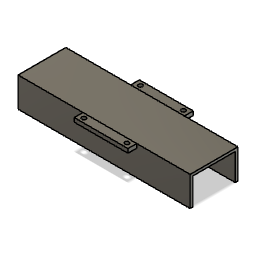
Magnet_Storage_Cover (Autodesk Fusion 360 design; units mm, degrees)
Autodesk Fusion 360 part; units mm, degrees
sketch "base" plane through (0, 0, 0) normal (0, 1, 0) x (1, 0, 0)
  line L0 (-67, 15.5) -> (67, 15.5) construction
  line L1 (67, 15.5) -> (67, -15.5) construction
  line L2 (67, -15.5) -> (-67, -15.5) construction
  line L3 (-67, -15.5) -> (-67, 15.5) construction
  line L4 (0, 15.5) -> (0, -15.5) construction
  line L5 (-67, 0) -> (67, 0) construction
  line L6 (-69.25, 17.75) -> (58.75, 17.75)
  line L7 (58.75, 17.75) -> (58.75, 15.75)
  line L8 (58.75, 15.75) -> (-69.25, 15.75)
  line L9 (-69.25, 15.75) -> (-69.25, 17.75)
  line L10 (-69.25, -15.75) -> (58.75, -15.75)
  line L11 (58.75, -15.75) -> (58.75, -17.75)
  line L12 (58.75, -17.75) -> (-69.25, -17.75)
  line L13 (-69.25, -17.75) -> (-69.25, -15.75)
  line L14 (-69.25, 15.75) -> (-69.25, -15.75)
  line L15 (-67.25, -15.75) -> (-67.25, 15.75)
  dimension "d1" = 134
  dimension "d2" = 31
  dimension "d3" = 128
  dimension "d4" = 2
  dimension "d5" = 2
  dimension "margin" = 0.25
  dimension "d7" = 0.25
  dimension "d8" = 0.25
  constraint horizontal L0
  constraint vertical L1
  constraint horizontal L2
  constraint vertical L3
  constraint midpoint L0 L4.start
  constraint midpoint L2 L4.end
  constraint midpoint L3 L5.start
  constraint midpoint L1 L5.end
  constraint coincident origin L5
  constraint coincident origin L4
  constraint horizontal L6
  constraint vertical L7
  constraint horizontal L8
  constraint vertical L9
  constraint horizontal L10
  constraint vertical L11
  constraint horizontal L12
  constraint vertical L13
  constraint collinear L7 L11
  constraint collinear L9 L13
  constraint coincident L10 L15.start
  constraint coincident L8 L15.end
  constraint perpendicular L8 L15
  constraint equal L9 L13
  measures "d1" distance of L0.start L0.end
  measures "d2" distance of L0.start L2.end
  measures "d3" distance of L6.start L6.end
  measures "d4" distance of L6.start L8.end
  measures "d5" distance of L14 L15
  measures "margin" distance of L3 L15
  measures "d7" distance of L2 L10
  measures "d8" distance of L0 L8
extrude "Extrude1" add sketch "base" along normal blind 20 makes body 1
sketch "top" plane through (0, 20, 0) normal (0, 1, 0) x (-1, 0, 0)
  line L0 (-58.75, 15.75) -> (67.25, 15.75)
  line L1 (67.25, 15.75) -> (67.25, -15.75)
  line L2 (67.25, -15.75) -> (-58.75, -15.75)
  line L3 (-58.75, -15.75) -> (-58.75, -17.75)
  line L4 (-58.75, -17.75) -> (69.25, -17.75)
  line L5 (69.25, -17.75) -> (69.25, 17.75)
  line L6 (69.25, 17.75) -> (-58.75, 17.75)
  line L7 (-58.75, 17.75) -> (-58.75, 15.75)
  line L8 (69.25, -17.75) -> (-58.75, -17.75)
  line L9 (-58.75, -17.75) -> (-58.75, 17.75)
  line L10 (-58.75, 17.75) -> (69.25, 17.75)
  line L11 (69.25, 17.75) -> (69.25, -17.75)
  constraint horizontal L8
  constraint vertical L9
  constraint horizontal L10
  constraint vertical L11
  constraint collinear L3 L9
  constraint collinear L5 L11
  constraint collinear L4 L8
  constraint collinear L6 L10
extrude "Extrude2" add sketch "top" along normal blind 2 bodies 1
sketch "wing supports" plane through (0, 22, 0) normal (0, 1, 0) x (-1, 0, 0)
  line L0 (69.25, 17.75) -> (-58.75, 17.75)
  line L1 (-58.75, 17.75) -> (-58.75, -17.75)
  line L2 (-58.75, -17.75) -> (69.25, -17.75)
  line L3 (69.25, -17.75) -> (69.25, 17.75)
  line L4 (21, -24.25) -> (-19, -24.25)
  line L5 (-19, -24.25) -> (-19, -17.75)
  line L6 (-19, -17.75) -> (21, -17.75)
  line L7 (21, -17.75) -> (21, -24.25)
  line L8 (21, 17.75) -> (-19, 17.75)
  line L9 (-19, 17.75) -> (-19, 24.25)
  line L10 (-19, 24.25) -> (21, 24.25)
  line L11 (21, 24.25) -> (21, 17.75)
  circle A0 centre (17, 21) radius 1.55
  circle A1 centre (-15, 21) radius 1.55
  line L12 (17, 21) -> (-15, 21) construction
  circle A2 centre (17, -21) radius 1.55
  circle A3 centre (-15, -21) radius 1.55
  line L13 (17, -21) -> (-15, -21) construction
  circle A4 centre (17, 21) radius 2.75
  circle A5 centre (-15, 21) radius 2.75
  circle A6 centre (17, -21) radius 2.75
  circle A7 centre (-15, -21) radius 2.75
  dimension "d13" = 6.5
  dimension "d14" = 40
  dimension "d15" = 19
  dimension "d16" = 3.1
  dimension "d17" = 3.25
  dimension "d18" = 4
  dimension "d19" = 4
  dimension "d20" = 3.25
  dimension "d21" = 4
  dimension "d22" = 4
  dimension "d25" = 5.5
  constraint horizontal L4
  constraint vertical L5
  constraint horizontal L6
  constraint vertical L7
  constraint horizontal L8
  constraint vertical L9
  constraint horizontal L10
  constraint vertical L11
  constraint collinear L5 L9
  constraint collinear L7 L11
  constraint collinear L2 L6
  constraint collinear L0 L8
  constraint equal L5 L9
  constraint equal A0 A1
  constraint coincident A0.centre L12.start
  constraint coincident A1.centre L12.end
  constraint horizontal L12
  constraint equal A2 A3
  constraint equal A0 A2
  constraint coincident A2.centre L13.start
  constraint coincident A3.centre L13.end
  constraint parallel L4 L13
  constraint concentric A1 A5
  constraint equal A4 A5
  constraint equal A4 A6
  constraint equal A4 A7
  measures "d13" distance of L4.end L5.end
  measures "d14" distance of L9.end L10.end
  measures "d15" distance of L5 origin
  measures "d16" diameter of A0
  measures "d17" distance of L10 L12
  measures "d18" distance of L11 A0.centre
  measures "d19" distance of L9 A1.centre
  measures "d20" distance of L4 L13
  measures "d21" distance of L7 A2.centre
  measures "d22" distance of L5 A3.centre
  measures "d25" diameter of A4
extrude "Extrude3" add sketch "wing supports" against normal blind 3 separate body contours L0 L8 L9 L10 L11 | L2 L4 L5 L6 L7 | A4 | A5 | A6 | A7 makes body 2 at (18.1833, 22, -21) makes body 3 at (18.1833, 22, 21)
extrude "Extrude4" [suppressed]
equation "d5 = d4"
equation "d7 = margin"
equation "d8 = margin"
equation "d19 = d18"
equation "d20 = d17"
equation "d21 = d18"
equation "d22 = d18"
